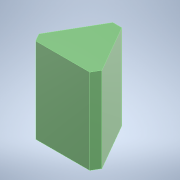
# Autodesk Inventor part: FactionSpecial_Council_CommandToken
Saved by Autodesk Inventor 2021 (Build 250183000, 183)
## iProperties
Created: 2023-03-16
Part Number: FactionSpecial_Council_CommandToken
Material: ABS Plastic
Document SubType Name: Modeling
Designer: Bradley
Density: 1.06 g/cm^3
Appearance: Smooth - Dark Forest Green
Author: Bradley
Autodesk Inventor part; units mm, degrees
ref_plane "YZ Plane" through (0, 0, 0) normal (1, 0, 0) x (0, 1, 0)
ref_plane "XZ Plane" through (0, 0, 0) normal (0, 1, 0) x (-1, 0, 0)
ref_plane "XY Plane" through (0, 0, 0) normal (0, 0, 1) x (1, 0, 0)
sketch "Sketch1" plane through (0, 0, 0) normal (0, 1, 0) x (-1, 0, 0)
  line L0 (1.6, -12.1429) -> (-1.6, -12.1429)
  line L1 (-1.6, -12.1429) -> (-11.3161, 4.6858)
  line L2 (-11.3161, 4.6858) -> (-9.7161, 7.4571)
  line L3 (-9.7161, 7.4571) -> (9.7161, 7.4571)
  line L4 (9.7161, 7.4571) -> (11.3161, 4.6858)
  line L5 (11.3161, 4.6858) -> (1.6, -12.1429)
  circle A0 centre (0, 0) radius 7.4571 construction
  dimension "d0" = 19.6
  dimension "d1" = 3.2
  dimension "d4" = 14.9142
  constraints: 12 end point, 4 equal length, 3 parallel, 3 tangent, 1 centre point, 1 coincident, 1 horizontal
  measures "d0" distance between parallel lines of L2 L5
  measures "d1" distance of L0.start L0.end
  measures "d4" diameter of A0
extrude "Extrusion1" add sketch "Sketch1" along normal mid plane 30.6
body "Solid1"
